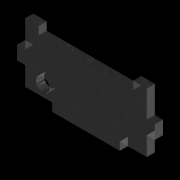
# Autodesk Inventor part: SideTopNM
Saved by Autodesk Inventor 2019 (Build 230136000, 136)
## iProperties
Created: 2019-05-08
Part Number: SideTopNM
Material: Acrylic, Clear
Document SubType Name: Modeling
Designer: super pig
Density: 1.19 g/cm^3
Appearance: Transparent - Clear
Mass: 3.1429 g
Surface Area: 22.6985 cm^2
Volume: 2.6411 cm^3
Name: Top Cover
Author: super pig
Autodesk Inventor part; units mm, degrees
ref_plane "YZ Plane" through (0, 0, 0) normal (1, 0, 0) x (0, 1, 0)
ref_plane "XZ Plane" through (0, 0, 0) normal (0, 1, 0) x (-1, 0, 0)
ref_plane "XY Plane" through (0, 0, 0) normal (0, 0, 1) x (1, 0, 0)
sketch "Sketch1" plane through (0, 0, 0) normal (0, 0, 1) x (1, 0, 0)
  line L0 (10, 3) -> (35, 3) projected
  line L1 (10, 0) -> (10, 3) projected
  line L2 (35, 0) -> (10, 0) projected
  line L3 (35, 0) -> (35, 3) projected
  line L4 (0, 3) -> (10, 3) projected
  line L5 (-3, 10) -> (-3, 15) projected
  line L6 (0, 15) -> (-3, 15) projected
  line L7 (0, 15) -> (0, 25) projected
  line L8 (35, 3) -> (45, 3) projected
  line L9 (45, 10) -> (45, 0) projected
  line L10 (48, 10) -> (45, 10) projected
  line L11 (48, 15) -> (48, 10) projected
  line L12 (45, 15) -> (48, 15) projected
  line L13 (45, 25) -> (45, 15) projected
  line L14 (0, 25) -> (5, 25)
  line L15 (5, 25) -> (5, 22)
  line L16 (5, 22) -> (0, 22)
  line L17 (0, 22) -> (0, 25)
  line L18 (45, 25) -> (40, 25)
  line L19 (40, 25) -> (40, 22)
  line L20 (40, 22) -> (45, 22)
  line L21 (45, 22) -> (45, 25)
  line L22 (5, 22) -> (40, 22)
  circle A0 centre (6.5, 7) radius 4 projected
  circle A1 centre (6.5, 7) radius 2.5
  line L23 (0, 10) -> (-3, 10) projected
  line L24 (0, 0) -> (0, 10) projected
  dimension "d0" = 5
  dimension "d1" = 3
  dimension "d2" = 5
  dimension "d3" = 3
  dimension "d4" = 5
  constraints: 18 end point, 4 parallel, 2 horizontal, 2 perpendicular, 2 point on line, 1 centre point, 1 coincident
  measures "d0" distance of L15.end L16.end
  measures "d1" distance of L14.end L15.end
  measures "d2" distance of L20.end L19.end
  measures "d3" distance of L19.end L18.end
  measures "d4" diameter of A1
extrude "Extrusion1" add sketch "Sketch1" along normal blind 3 contours A0 | L4 L24 L23 L5 L6 L7 L16 L22 L20 L13 L12 L11 L10 L9 L8 L0 | L0 L3 L2 L1 | L20 L19 L18 L13 | L7 L14 L15 L16
body "Solid1"
